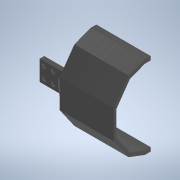
# Autodesk Inventor part: krilo
Saved by Autodesk Inventor 2022 (Build 260153000, 153)
## iProperties
Created: 2023-04-21
Part Number: krilo
Material: Типовые
Document SubType Name: Modeling
Designer: korsh624
Density: 1 g/cm^3
Appearance: Темно-серый
Author: korsh624
Autodesk Inventor part; units mm, degrees
ref_plane "YZ Plane" through (0, 0, 0) normal (1, 0, 0) x (0, 1, 0)
ref_plane "XZ Plane" through (0, 0, 0) normal (0, 1, 0) x (-1, 0, 0)
ref_plane "XY Plane" through (0, 0, 0) normal (0, 0, 1) x (1, 0, 0)
sketch "Эскиз1" plane through (0, 0, 0) normal (0, 0, 1) x (1, 0, 0)
  circle A0 centre (10.1, 79.7047) radius 2 projected
  circle A1 centre (26.1, 79.7047) radius 2 projected
  circle A2 centre (26.1, 60.2954) radius 2 projected
  circle A3 centre (10.1, 60.2954) radius 2 projected
  line L0 (55.6, -87.7197) -> (55.6, 87.7197) projected
  line L1 (2.7744, 52.2954) -> (55.6, 52.2954)
  line L2 (55.6, 52.2954) -> (55.6, 87.7197)
  line L3 (55.6, 87.7197) -> (2.7744, 87.7197)
  line L4 (2.7744, 87.7197) -> (2.7744, 52.2954)
  point P0 (0, 0)
  dimension "d0" = 8.0151
  dimension "d1" = 8
  constraints: 8 end point, 2 parallel, 1 horizontal, 1 perpendicular
  measures "d0" distance from line of L3 A0.centre
  measures "d1" distance from line of L1 A3.centre
extrude "Выдавливание1" add sketch "Эскиз1" along normal blind 8
sketch "Эскиз2" plane through (0, 0, 8) normal (0, 0, 1) x (1, 0, 0)
  circle A0 centre (10.1, 79.7047) radius 2 projected
  circle A1 centre (26.1, 79.7047) radius 2 projected
  circle A2 centre (26.1, 60.2954) radius 2 projected
  circle A3 centre (10.1, 60.2954) radius 2 projected
  line L0 (14.4301, 79.7047) -> (12.2651, 75.9547)
  line L1 (12.2651, 75.9547) -> (7.9349, 75.9547)
  line L2 (7.9349, 75.9547) -> (5.7699, 79.7047)
  line L3 (5.7699, 79.7047) -> (7.9349, 83.4547)
  line L4 (7.9349, 83.4547) -> (12.2651, 83.4547)
  line L5 (12.2651, 83.4547) -> (14.4301, 79.7047)
  line L6 (21.7699, 79.7047) -> (23.9349, 83.4547)
  line L7 (23.9349, 83.4547) -> (28.2651, 83.4547)
  line L8 (28.2651, 83.4547) -> (30.4301, 79.7047)
  line L9 (30.4301, 79.7047) -> (28.2651, 75.9547)
  line L10 (28.2651, 75.9547) -> (23.9349, 75.9547)
  line L11 (23.9349, 75.9547) -> (21.7699, 79.7047)
  line L12 (21.7699, 60.2954) -> (23.9349, 64.0454)
  line L13 (23.9349, 64.0454) -> (28.2651, 64.0454)
  line L14 (28.2651, 64.0454) -> (30.4301, 60.2954)
  line L15 (30.4301, 60.2954) -> (28.2651, 56.5454)
  line L16 (28.2651, 56.5454) -> (23.9349, 56.5454)
  line L17 (23.9349, 56.5454) -> (21.7699, 60.2954)
  line L18 (14.4301, 60.2954) -> (12.2651, 56.5454)
  line L19 (12.2651, 56.5454) -> (7.9349, 56.5454)
  line L20 (7.9349, 56.5454) -> (5.7699, 60.2954)
  line L21 (5.7699, 60.2954) -> (7.9349, 64.0454)
  line L22 (7.9349, 64.0454) -> (12.2651, 64.0454)
  line L23 (12.2651, 64.0454) -> (14.4301, 60.2954)
  point P0 (0, 0)
  dimension "d4" = 7.5
  dimension "d5" = 7.5
  dimension "d6" = 7.5
  dimension "d7" = 7.5
  constraints: 48 end point, 4 coincident, 52 other
  measures "d4" distance between parallel lines of L1 L4
  measures "d5" distance between parallel lines of L10 L7
  measures "d6" distance between parallel lines of L16 L13
  measures "d7" distance between parallel lines of L22 L19
extrude "Выдавливание2" cut sketch "Эскиз2" against normal blind 4
sketch "Эскиз3" plane through (55.6, 52.2954, 0) normal (1, 0, 0) x (0, 0, -1)
  line L0 (0, 35.4244) -> (-8, 35.4244) projected
  line L1 (0, 0) -> (-8, 0) projected
  line L2 (0, 35.4244) -> (0, 0) projected
  line L3 (0, 17.7122) -> (-25.9453, 17.7122)
  line L4 (-25.9453, 17.7122) -> (-25.9453, 42.7122)
  line L5 (-25.9453, 42.7122) -> (0, 79.5939)
  line L6 (0, 79.5939) -> (28.389, 90.3911)
  line L7 (28.389, 90.3911) -> (38.389, 90.3911)
  line L8 (38.389, 90.3911) -> (38.389, 83.3911)
  line L9 (38.389, 83.3911) -> (28.389, 83.3911)
  line L10 (28.389, 83.3911) -> (2.3259, 73.4785)
  line L11 (2.3259, 73.4785) -> (-21.5116, 39.5932)
  line L12 (-21.5116, 39.5932) -> (-21.5116, 17.7122)
  line L13 (0, 0) -> (-8, 0)
  line L14 (-25.9453, 17.7122) -> (-25.9453, -7.2878)
  line L15 (-25.9453, -7.2878) -> (0, -44.1695)
  line L16 (0, -44.1695) -> (28.389, -54.9667)
  line L17 (28.389, -54.9667) -> (38.389, -54.9667)
  line L18 (38.389, -54.9667) -> (38.389, -47.9667)
  line L19 (38.389, -47.9667) -> (28.389, -47.9667)
  line L20 (28.389, -47.9667) -> (2.3259, -38.0541)
  line L21 (2.3259, -38.0541) -> (-21.5116, -4.1688)
  line L22 (-21.5116, -4.1688) -> (-21.5116, 17.7122)
  line L23 (0, 35.4244) -> (-8, 35.4244) projected
  line L24 (0, 35.4244) -> (-21.5116, 35.4244)
  line L25 (-21.5116, 35.4244) -> (-21.5116, 0)
  line L26 (-21.5116, 0) -> (0, 0)
  line L27 (0, 0) -> (0, 35.4244)
  point P0 (0, -52.2954)
  dimension "d10" = 25
  dimension "d11" = 10
  dimension "d12" = 7
  constraints: 48 end point, 8 symmetric about line, 4 perpendicular, 3 parallel, 2 horizontal, 2 point on line, 1 midpoint, 1 vertical
  measures "d10" distance of L3.end L4.end
  measures "d11" distance of L6.end L7.end
  measures "d12" distance of L7.end L8.end
extrude "Выдавливание3" add sketch "Эскиз3" along normal blind 15
sketch "Эскиз4" plane through (70.6, 52.2954, 0) normal (1, 0, 0) x (0, 0, -1)
  line L0 (-21.5116, 0) -> (0, 0) projected
  line L1 (0, 0) -> (0, 35.4244) projected
  line L2 (0, 35.4244) -> (-21.5116, 35.4244) projected
  line L3 (-21.5116, 35.4244) -> (-21.5116, 39.5932) projected
  line L4 (-21.5116, 39.5932) -> (2.3259, 73.4785) projected
  line L5 (2.3259, 73.4785) -> (28.389, 83.3911) projected
  line L6 (28.389, 83.3911) -> (38.389, 83.3911) projected
  line L7 (38.389, 83.3911) -> (38.389, 90.3911) projected
  line L8 (38.389, 90.3911) -> (28.389, 90.3911) projected
  line L9 (28.389, 90.3911) -> (0, 79.5939) projected
  line L10 (0, 79.5939) -> (-25.9453, 42.7122) projected
  line L11 (-25.9453, 42.7122) -> (-25.9453, -7.2878) projected
  line L12 (-25.9453, -7.2878) -> (0, -44.1695) projected
  line L13 (0, -44.1695) -> (28.389, -54.9667) projected
  line L14 (28.389, -54.9667) -> (38.389, -54.9667) projected
  line L15 (38.389, -54.9667) -> (38.389, -47.9667) projected
  line L16 (38.389, -47.9667) -> (28.389, -47.9667) projected
  line L17 (28.389, -47.9667) -> (2.3259, -38.0541) projected
  line L18 (2.3259, -38.0541) -> (-21.5116, -4.1688) projected
  line L19 (-21.5116, -4.1688) -> (-21.5116, 0) projected
  line L20 (-21.5116, 0) -> (-8, 0) projected
  line L21 (0, 35.4244) -> (-21.5116, 35.4244) projected
  line L22 (-21.5116, 0) -> (-21.5116, 35.4244)
  point P0 (0, -52.2954)
  constraints: 2 end point, 1 vertical
extrude "Выдавливание4" add sketch "Эскиз4" along normal blind 80 contours L19 L18 L17 L16 L15 L14 L13 L12 L11 L10 L9 L8 L7 L6 L5 L4 L3 L22
sketch "Эскиз5" plane through (55.6, 52.2954, 0) normal (-1, 0, 0) x (0, 0, 1)
  line L0 (8, 0) -> (8, 35.4244) projected
  line L1 (25.9453, 42.7122) -> (25.9453, -7.2878) projected
  line L2 (8, 22.7122) -> (25.9453, 22.7122)
  line L3 (25.9453, 22.7122) -> (25.9453, 12.7122)
  line L4 (25.9453, 12.7122) -> (8, 12.7122)
  line L5 (8, 12.7122) -> (8, 22.7122)
  line L6 (21.5116, 0) -> (8, 0) projected
  line L7 (8, 35.4244) -> (21.5116, 35.4244) projected
  point P0 (0, -52.2954)
  point P1 (8, 12.7122)
  point P2 (25.9453, 22.7122)
  dimension "d17" = 10
  dimension "d18" = 35.4244
  dimension "d19" = 12.7122
  constraints: 8 end point, 2 parallel, 2 point on line, 1 horizontal, 1 perpendicular
  measures "d17" distance of L2.end L3.end
  measures "d18" distance between parallel lines of L6 L7
  measures "d19" distance between parallel lines of L7 L2
extrude "Выдавливание5" add sketch "Эскиз5" along normal blind 20
sketch "Эскиз6" plane through (55.6, 65.0076, 8) normal (0, -1, 0) x (1, 0, 0)
  line L0 (0, 17.9453) -> (0, 0) projected
  line L1 (0, 17.9453) -> (-20, 17.9453) projected
  line L2 (-20, 0) -> (-20, 17.9453) projected
  line L3 (0, 0) -> (-20, 0) projected
  line L4 (0, 17.9453) -> (0, -8) projected
  line L5 (-20, 0) -> (0, 17.9453)
  point P0 (-55.6, -8)
  constraints: 2 end point
extrude "Выдавливание6" cut sketch "Эскиз6" against normal blind 20 contours L5 L2 L1
fillet "Сопряжение1" radius 5 1 edges at (70.6, 70.0076, 21.5116)
sketch "Эскиз7" plane through (70.6, 52.2954, 0) normal (1, 0, 0) x (0, 0, -1)
  circle A0 centre (-14.7558, 29.0683) radius 3
  point P0 (0, -52.2954)
  constraints: 1 centre point, 2 other
extrude "Выдавливание7" cut sketch "Эскиз7" against normal blind 10
sketch "Эскиз8" plane through (70.6, 52.2954, 0) normal (1, 0, 0) x (0, 0, -1)
  circle A0 centre (-14.7558, 6.3561) radius 3
  point P0 (0, -52.2954)
  constraints: 1 centre point, 2 other
extrude "Выдавливание8" cut sketch "Эскиз8" against normal blind 10
equation "\"d5\" = d4"
equation "\"d6\" = d4"
equation "\"d7\" = d6"
equation "\"d19\" = -0.5 * d17 + 0.5 * d18"
